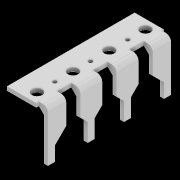
# Autodesk Inventor part: suporte 555
Saved by Autodesk Inventor 2020 (Build 240168000, 168)
## iProperties
Created: 2020-02-11
Part Number: suporte 555
Material: Generic
Document SubType Name: Modeling
Designer: PEDRO
Density: 1 g/cm^3
Appearance: Default
Author: PEDRO
Autodesk Inventor part; units mm, degrees
ref_plane "YZ Plane" through (0, 0, 0) normal (1, 0, 0) x (0, 1, 0)
sketch "Sketch1" plane through (0, 0, 0) normal (0, 1, 0) x (-1, 0, 0)
  line L0 (0, 0) -> (22.85, 0)
  line L1 (22.85, 0) -> (22.85, -100)
  line L2 (22.85, -100) -> (0, -100)
  line L3 (0, -100) -> (0, 0)
  circle A0 centre (7.12, -92.8) radius 4
  circle A1 centre (7.12, -64.4) radius 4
  circle A2 centre (7.12, -35.95) radius 4
  circle A3 centre (7.12, -7.71) radius 4
  circle A4 centre (7.12, -21.73) radius 1.5
  circle A5 centre (7.12, -49.67) radius 1.5
  circle A6 centre (7.12, -78.83) radius 1.5
  line L4 (7.12, -7.71) -> (-9.9799, -7.71) construction
  line L5 (7.12, -35.95) -> (-7.15, -35.95) construction
  line L6 (7.12, -64.4) -> (-7.15, -64.4) construction
  line L7 (7.12, -92.8) -> (-7.15, -92.8) construction
  line L8 (0, -27.427) -> (-7.15, -27.427)
  line L9 (0, -44.473) -> (-7.15, -44.473)
  line L10 (0, -55.877) -> (-7.15, -55.877)
  line L11 (0, -72.923) -> (-7.15, -72.923)
  line L12 (0, -84.277) -> (-7.15, -84.277)
  line L13 (0, -98.46) -> (-7.15, -98.46)
  line L14 (0, -2.05) -> (-7.15, -2.05)
  line L15 (0, -16.233) -> (-7.15, -16.233)
  line L16 (-7.15, -2.05) -> (-7.15, -16.233)
  line L17 (-7.15, -27.427) -> (-7.15, -44.473)
  line L18 (-7.15, -55.877) -> (-7.15, -72.923)
  line L19 (-7.15, -84.277) -> (-7.15, -98.46)
  line L20 (-7.15, 0) -> (-7.15, -100) construction
  dimension "d0" = 22.85
  dimension "d1" = 100
  dimension "d2" = 8
  dimension "d3" = 8
  dimension "d4" = 8
  dimension "d5" = 8
  dimension "d7" = 0
  dimension "d8" = 0
  dimension "d9" = 0
  dimension "d10" = 7.71
  dimension "d11" = 35.95
  dimension "d12" = 64.4
  dimension "d13" = 92.8
  dimension "d14" = 3
  dimension "d15" = 3
  dimension "d16" = 3
  dimension "d17" = 7.12
  dimension "d18" = 7.12
  dimension "d19" = 0
  dimension "d20" = 0
  dimension "d21" = 21.73
  dimension "d22" = 49.67
  dimension "d23" = 78.83
  dimension "d28" = 8.523
  dimension "d29" = 8.523
  dimension "d30" = 8.523
  dimension "d31" = 8.523
  dimension "d32" = 8.523
  dimension "d33" = 5.66
  dimension "d34" = 5.66
  dimension "d35" = 8.523
  dimension "d36" = 100
  dimension "d42" = 7.15
  constraints: 40 end point, 9 parallel, 7 centre point, 5 perpendicular, 4 point on line, 3 vertical, 2 collinear, 2 horizontal, 11 other
  measures "d0" distance of L1.end L2.end
  measures "d1" distance of L0.end L1.end
  measures "d2" diameter of A0
  measures "d3" diameter of A1
  measures "d4" diameter of A2
  measures "d5" diameter of A3
  measures "d7" horizontal distance of L4.start L5.start
  measures "d8" horizontal distance of L4.start L6.start
  measures "d9" horizontal distance of L4.start L7.start
  measures "d10" distance from line of L4.start L0
  measures "d11" distance from line of L5.start L0
  measures "d12" distance from line of L6.start L0
  measures "d13" distance from line of L0 L7.start
  measures "d14" diameter of A4
  measures "d15" diameter of A5
  measures "d16" diameter of A6
  measures "d19" horizontal distance of A4.centre A5.centre
  measures "d20" horizontal distance of A5.centre A6.centre
  measures "d21" distance from line of L0 A4.centre
  measures "d22" distance from line of L0 A5.centre
  measures "d23" distance from line of L0 A6.centre
  measures "d28" distance between parallel lines of L5 L8
  measures "d29" distance between parallel lines of L5 L9
  measures "d30" distance between parallel lines of L6 L10
  measures "d31" distance between parallel lines of L6 L11
  measures "d32" distance between parallel lines of L7 L12
  measures "d33" distance between parallel lines of L7 L13
  measures "d34" distance between parallel lines of L4 L14
  measures "d35" distance between parallel lines of L4 L15
  measures "d36" distance of L20.start L20.end
  measures "d42" distance of the line from the sketch origin of L20
extrude "Extrusion1" add sketch "Sketch1" against normal blind 3
ref_plane "Work Plane2" through (7.15, 0, -16.233) normal (1, 0, 0) x (0, 0, -1)
ref_plane "Work Plane3" through (7.15, 0, -2.05) normal (1, 0, 0) x (0, 0, -1)
sketch "Sketch3" plane through (7.15, 0, -2.05) normal (1, 0, 0) x (0, 0, -1)
  line L0 (0, 0) -> (14.183, 0) projected
  line L1 (14.183, -3) -> (0, -3) projected
  line L2 (14.183, 0) -> (14.183, -3) projected
  line L3 (0, 0) -> (0, -3) projected
  line L4 (25.377, 0) -> (42.423, 0) projected
  line L5 (25.377, 0) -> (25.377, -3) projected
  line L6 (42.423, -3) -> (25.377, -3) projected
  line L7 (42.423, 0) -> (42.423, -3) projected
  line L8 (53.827, 0) -> (70.873, 0) projected
  line L9 (53.827, 0) -> (53.827, -3) projected
  line L10 (70.873, -3) -> (53.827, -3) projected
  line L11 (70.873, 0) -> (70.873, -3) projected
  line L12 (82.227, 0) -> (96.41, 0) projected
  line L13 (82.227, 0) -> (82.227, -3) projected
  line L14 (96.41, -3) -> (82.227, -3) projected
  line L15 (96.41, 0) -> (96.41, -3) projected
  line L16 (0, 0) -> (0, -40)
  line L17 (0, -40) -> (5.4, -40)
  line L18 (14.183, 0) -> (14.183, -20)
  line L19 (5.4, -40) -> (5.4, -28.783)
  line L20 (14.183, -20) -> (5.4, -28.783)
  line L21 (96.41, 0) -> (96.41, -40)
  line L22 (96.41, -40) -> (91.01, -40)
  line L23 (82.227, 0) -> (82.227, -20)
  line L24 (91.01, -40) -> (91.01, -28.783)
  line L25 (82.227, -20) -> (91.01, -28.783)
  line L26 (70.873, 0) -> (70.873, -20)
  line L27 (53.827, 0) -> (53.827, -20)
  line L28 (70.873, -20) -> (65.05, -25.823)
  line L29 (65.05, -25.823) -> (65.05, -40)
  line L30 (65.05, -40) -> (59.65, -40)
  line L31 (59.65, -40) -> (59.65, -25.823)
  line L32 (59.65, -25.823) -> (53.827, -20)
  line L33 (62.35, -40) -> (62.35, 0) construction
  line L34 (53.827, 0) -> (70.873, 0) projected
  line L35 (42.423, 0) -> (42.423, -20)
  line L36 (25.377, 0) -> (25.377, -20)
  line L37 (42.423, -20) -> (36.6, -25.823)
  line L38 (36.6, -25.823) -> (36.6, -40)
  line L39 (36.6, -40) -> (31.2, -40)
  line L40 (31.2, -40) -> (31.2, -25.823)
  line L41 (31.2, -25.823) -> (25.377, -20)
  line L42 (33.9, -40) -> (33.9, 0) construction
  point P0 (82.227, -3)
  dimension "d46" = 40
  dimension "d47" = 5.4
  dimension "d48" = 20
  dimension "d51" = 135
  dimension "d56" = 135
  dimension "d57" = 5.4
  dimension "d58" = 40
  dimension "d59" = 20
  dimension "d61" = 20
  dimension "d62" = 135
  dimension "d63" = 135
  dimension "d64" = 5.4
  dimension "d66" = 20
  dimension "d67" = 20
  dimension "d68" = 135
  dimension "d69" = 135
  dimension "d70" = 5.4
  dimension "d71" = 20
  constraints: 52 end point, 9 vertical, 8 perpendicular, 6 collinear, 4 midpoint, 1 horizontal, 1 other
  measures "d46" distance of L0.start L16.end
  measures "d47" distance of L16.end L17.end
  measures "d48" distance of L0.end L18.end
  measures "d51" angle of L18 L20
  measures "d56" angle of L25 L23
  measures "d57" distance of L21.end L24.start
  measures "d58" distance of L12.end L21.end
  measures "d59" distance of L23.start L23.end
  measures "d61" distance of L8.end L26.end
  measures "d62" angle of L27 L32
  measures "d63" angle of L26 L28
  measures "d64" distance of L29.end L30.end
  measures "d66" distance of L8.start L27.end
  measures "d67" distance of L4.end L35.end
  measures "d68" angle of L36 L41
  measures "d69" angle of L35 L37
  measures "d70" distance of L39.start L39.end
  measures "d71" distance of L4.start L41.end
extrude "Extrusion2" add sketch "Sketch3" against normal blind 3
fillet "Fillet1" radius 4 4 edges at (7.15, 0, -9.1415) (7.15, 0, -35.95) (7.15, 0, -64.4) (7.15, 0, -91.3685)
chamfer "Chamfer1" distance 4 angle 45 4 edges at (4.15, -3, -9.1415) (4.15, -3, -35.95) (4.15, -3, -64.4) (4.15, -3, -91.3685)
equation "\"d18\" = d17"
equation "\"d57\" = d47"
equation "\"d58\" = d46"
equation "\"d59\" = d48"
body "Solid1"
